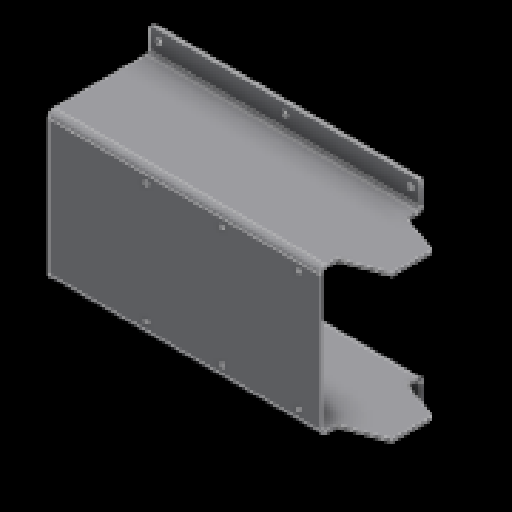
# Autodesk Inventor part: PowerSupplyMount
Saved by Autodesk Inventor 2025.2 (Build 292293000, 293)
## iProperties
Created: 2025-11-18
Part Number: PowerSupplyMount
Material: Generic
Document SubType Name: Sheet Metal
Designer: valer
Density: 1 g/cm^3
Sheet Metal Rule: Default
Appearance: Default
Author: valer
Autodesk Inventor part; units mm, degrees
ref_plane "YZ Plane" through (0, 0, 0) normal (1, 0, 0) x (0, 1, 0)
ref_plane "XZ Plane" through (0, 0, 0) normal (0, 1, 0) x (-1, 0, 0)
ref_plane "XY Plane" through (0, 0, 0) normal (0, 0, 1) x (1, 0, 0)
sketch "Base" plane through (0, 0, 0) normal (1, 0, 0) x (0, 1, 0)
  line L0 (98, 0) -> (73, 0)
  line L1 (73, 0) -> (73, 100)
  line L2 (73, 100) -> (0, 100)
  line L3 (0, -20) -> (0, 120) construction
  line L4 (-137.2, 0) -> (137.2, 0) construction
  line L5 (-98, 0) -> (-73, 0)
  line L6 (-73, 0) -> (-73, 100)
  line L7 (-73, 100) -> (0, 100)
  point P0 (0, 0)
  dimension "d0" = 25
  dimension "d1" = 100
  dimension "d2" = 73
  measures "d0" distance of L0.start L0.end
  measures "d1" distance of L0.end L1.end
  measures "d2" distance of L1.end L2.end
contour flange "BaseFeature" sketch "Base" thickness 3 bend radius 3 width 270 along (1, 0, 0) mid plane no both sides no wall seen from (0, -85.5, 0) lies toward (0, 0, -1) curves L5 L6 L7 L2 L1 L0
bend "Bend1"
corner "Corner1"
sketch "BodyMountHoles" plane through (0, 76, 0) normal (0, 0, 1) x (1, 0, 0)
  line L0 (-59.4, -76) -> (356.4, -76) construction
  line L1 (0, 22) -> (270, 22) construction
  line L2 (135, 22) -> (135, -174) construction
  line L3 (0, -174) -> (270, -174) construction
  circle A0 centre (260, 12) radius 3
  line L4 (270, 22) -> (270, 0) projected
  circle A1 centre (135, 12) radius 3
  line L5 (135, 12) -> (260, 12) construction
  circle A2 centre (10, 12) radius 3
  circle A3 centre (260, -164) radius 3
  circle A4 centre (135, -164) radius 3
  circle A5 centre (10, -164) radius 3
  point P0 (0, -76)
  dimension "d14" = 6
  dimension "d15" = 10
  dimension "d16" = 10
  constraints: 6 centre point, 4 end point, 4 symmetric about line, 2 midpoint, 1 equal radius, 1 horizontal, 1 point on line, 4 other
  measures "d14" diameter of A0
  measures "d15" distance from line of L1 L5.end
  measures "d16" distance from line of L4 L5.end
extrude "BodyMountHolesFeature" cut sketch "BodyMountHoles" against normal blind 3
fillet "FilletsFeature" radius 4 4 edges at (0, 98, -1.5) (270, 98, -1.5) (0, -98, -1.5) (270, -98, -1.5)
sketch "ConverterMountHoles" plane through (0, 67, 100) normal (0, 0, 1) x (1, 0, 0)
  arc A0 (250.95, -126.5) -> (245.95, -126.5) centre (248.45, -126.5) ccw construction
  line L0 (61.45, -122) -> (284.45, -122) construction
  line L1 (284.45, -122) -> (284.45, -132) construction
  line L2 (284.45, -132) -> (250.95, -132) construction
  line L3 (250.95, -132) -> (250.95, -126.5) construction
  arc A1 (250.95, -126.5) -> (245.95, -126.5) centre (248.45, -126.5) ccw construction
  line L4 (245.95, -126.5) -> (245.95, -132) construction
  line L5 (245.95, -132) -> (175.45, -132) construction
  line L6 (175.45, -132) -> (175.45, -126.5) construction
  arc A2 (175.45, -126.5) -> (170.45, -126.5) centre (172.95, -126.5) ccw construction
  line L7 (170.45, -126.5) -> (170.45, -132) construction
  line L8 (170.45, -132) -> (99.95, -132) construction
  line L9 (99.95, -132) -> (99.95, -126.5) construction
  arc A3 (99.95, -126.5) -> (94.95, -126.5) centre (97.45, -126.5) ccw construction
  line L10 (94.95, -126.5) -> (94.95, -132) construction
  line L11 (94.95, -132) -> (61.45, -132) construction
  line L12 (61.45, -132) -> (61.45, -122) construction
  line L13 (284.45, -12) -> (61.45, -12) construction
  line L14 (61.45, -12) -> (61.45, -2) construction
  line L15 (61.45, -2) -> (94.95, -2) construction
  line L16 (94.95, -2) -> (94.95, -7.5) construction
  arc A4 (94.95, -7.5) -> (99.95, -7.5) centre (97.45, -7.5) ccw construction
  line L17 (99.95, -7.5) -> (99.95, -2) construction
  line L18 (99.95, -2) -> (170.45, -2) construction
  line L19 (170.45, -2) -> (170.45, -7.5) construction
  arc A5 (170.45, -7.5) -> (175.45, -7.5) centre (172.95, -7.5) ccw construction
  line L20 (175.45, -7.5) -> (175.45, -2) construction
  line L21 (175.45, -2) -> (245.95, -2) construction
  line L22 (245.95, -2) -> (245.95, -7.5) construction
  arc A6 (245.95, -7.5) -> (250.95, -7.5) centre (248.45, -7.5) ccw construction
  line L23 (250.95, -7.5) -> (250.95, -2) construction
  line L24 (250.95, -2) -> (284.45, -2) construction
  line L25 (284.45, -2) -> (284.45, -12) construction
  circle A7 centre (248.45, -126.5) radius 2
  circle A8 centre (172.95, -126.5) radius 2
  circle A9 centre (97.45, -126.5) radius 2
  circle A10 centre (248.45, -7.5) radius 2
  circle A11 centre (172.95, -7.5) radius 2
  circle A12 centre (97.45, -7.5) radius 2
  point P0 (0, -67)
  dimension "d20" = 4
  constraints: 6 centre point, 6 coincident, 5 equal radius
  measures "d20" diameter of A7
extrude "ConverterMountHolesFeature" cut sketch "ConverterMountHoles" against normal blind 3
sketch "Sketch4" plane through (0, 73, 3) normal (0, 1, 0) x (1, 0, 0)
  line L0 (270, 0) -> (270, -91)
  line L1 (270, -10) -> (302, -10)
  line L2 (302, -10) -> (302, -45)
  line L3 (302, -45) -> (270, -77)
  line L4 (270, -91) -> (270, 0)
  point P0 (0, 3)
  dimension "d23" = 32
  dimension "d26" = 35
  dimension "d32" = 10
  dimension "d33" = 45
  measures "d23" distance between parallel lines of L4 L2
  measures "d26" distance of L1.end L2.end
  measures "d32" distance from line of L1 L0.start
  measures "d33" angle of L0 L3
sheet face with bend "Face1" sketch "Sketch4" thickness 3 toward (0, -1, 0) bend radius 3
bend "Bend2"
mirror "Mirror1" about plane through (0, 0, 0) normal (0, 1, 0)
fillet "Fillet2" radius 4 8 edges at (302, 71.5, 13) (302, -71.5, 13) (302, -71.5, 48) (302, 71.5, 48) (270, 71.5, 80) (270, -71.5, 80) (270, 71.5, 13) (270, -71.5, 13)
sketch "Sketch6" plane through (0, 73, 3) normal (0, 1, 0) x (1, 0, 0)
  circle A0 centre (295, -19) radius 2 projected
  circle A1 centre (30, -6.3) radius 2 projected
  circle A2 centre (30, -31.7) radius 2 projected
  point P0 (0, 3)
extrude "Cut3" cut sketch "Sketch6" against normal through all
equation "\"d17\" = Thickness"
equation "\"d21\" = Thickness"
equation "\"d35\" = Thickness"
equation "\"d3\" = Thickness"
equation "\"d4\" = BendReliefWidth"
equation "\"d5\" = BendReliefDepth"
equation "\"d6\" = MinimumRemnant"
equation "\"d7\" = TransitionRadius"
equation "\"d9\" = BendRadius"
equation "\"d11\" = CornerReliefSize"
equation "\"d12\" = GapSize"
equation "\"d13\" = JacobiRadiusSize"
equation "\"d27\" = BendRadius"
equation "\"d28\" = BendReliefWidth"
equation "\"d30\" = MinimumRemnant"
equation "\"d29\" = BendReliefDepth"
equation "\"d31\" = TransitionRadius"
equation "\"BendRadius\" = Thickness"
equation "\"BendReliefWidth\" = Thickness"
equation "\"BendReliefDepth\" = 0.5 * Thickness"
equation "\"CornerReliefSize\" = 4 * Thickness"
equation "\"MinimumRemnant\" = 2 * Thickness"
equation "\"TransitionRadius\" = BendRadius"
equation "\"JacobiRadiusSize\" = BendRadius"
equation "\"GapSize\" = Thickness"
equation "\"Thickness\" = 3"
body "Solid1"
